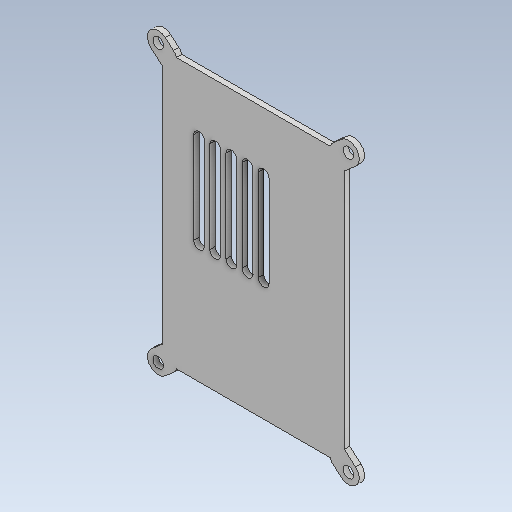
# Autodesk Inventor part: Case Cover Rev D
Saved by Autodesk Inventor 2021 (Build 250183000, 183)
## iProperties
Created: 2021-07-31
Part Number: Case Cover Rev D
Material: Generic
Document SubType Name: Modeling
Designer: cmzgt
Density: 1 g/cm^3
Appearance: Default
Author: cmzgt
Autodesk Inventor part; units mm, degrees
ref_plane "YZ Plane" through (0, 0, 0) normal (1, 0, 0) x (0, 1, 0)
ref_plane "XZ Plane" through (0, 0, 0) normal (0, 1, 0) x (-1, 0, 0)
ref_plane "XY Plane" through (0, 0, 0) normal (0, 0, 1) x (1, 0, 0)
sketch "Sketch1" plane through (0, 0, 0) normal (0, 0, 1) x (1, 0, 0)
  circle A0 centre (35.3094, -51.3621) radius 1.985 projected
  circle A1 centre (-35.3094, -51.3621) radius 1.985 projected
  circle A2 centre (-35.3094, 51.3621) radius 1.985 projected
  circle A3 centre (35.3094, 51.3621) radius 1.985 projected
  line L0 (28.5119, 50.05) -> (-28.5119, 50.05) projected
  arc A4 (-28.5119, 50.05) -> (-29.6663, 51.7567) centre (-32.2906, 48.7379) ccw projected
  line L1 (-32.6852, 54.381) -> (-29.6663, 51.7567) projected
  arc A5 (-32.6852, 54.381) -> (-37.9337, 48.3433) centre (-35.3094, 51.3621) ccw projected
  line L2 (-33.8, 44.7499) -> (-37.9337, 48.3433) projected
  line L3 (-33.8, 44.7499) -> (-33.8, -44.7499) projected
  line L4 (-37.9337, -48.3433) -> (-33.8, -44.7499) projected
  arc A6 (-37.9337, -48.3433) -> (-32.6852, -54.381) centre (-35.3094, -51.3621) ccw projected
  line L5 (-29.6663, -51.7567) -> (-32.6852, -54.381) projected
  arc A7 (-29.6663, -51.7567) -> (-28.5119, -50.05) centre (-32.2906, -48.7379) ccw projected
  line L6 (-28.5119, -50.05) -> (28.5119, -50.05) projected
  arc A8 (28.5119, -50.05) -> (29.6663, -51.7567) centre (32.2906, -48.7379) ccw projected
  line L7 (32.6852, -54.381) -> (29.6663, -51.7567) projected
  arc A9 (32.6852, -54.381) -> (37.9337, -48.3433) centre (35.3094, -51.3621) ccw projected
  line L8 (33.8, -44.7499) -> (37.9337, -48.3433) projected
  line L9 (33.8, -44.7499) -> (33.8, 44.7499) projected
  line L10 (37.9337, 48.3433) -> (33.8, 44.7499) projected
  arc A10 (37.9337, 48.3433) -> (32.6852, 54.381) centre (35.3094, 51.3621) ccw projected
  line L11 (29.6663, 51.7567) -> (32.6852, 54.381) projected
  arc A11 (29.6663, 51.7567) -> (28.5119, 50.05) centre (32.2906, 48.7379) ccw projected
  line L12 (-30.6, -44.85) -> (-30.6, 44.85) projected
  arc A12 (-28.6, 46.85) -> (-30.6, 44.85) centre (-28.6, 44.85) ccw projected
  line L13 (-28.6, 46.85) -> (28.6, 46.85) projected
  arc A13 (30.6, 44.85) -> (28.6, 46.85) centre (28.6, 44.85) ccw projected
  line L14 (30.6, 44.85) -> (30.6, -44.85) projected
  arc A14 (28.6, -46.85) -> (30.6, -44.85) centre (28.6, -44.85) ccw projected
  line L15 (28.6, -46.85) -> (-28.6, -46.85) projected
  arc A15 (-30.6, -44.85) -> (-28.6, -46.85) centre (-28.6, -44.85) ccw projected
  point P0 (0, 0)
extrude "Extrusion1" add sketch "Sketch1" along normal blind 2 contours A11 L11 A10 L10 L9 L8 A9 L7 A8 L6 A7 L5 A6 L4 L3 L2 A5 L1 A4 L0 | L12 A12 L13 A13 L14 A14 L15 A15
sketch "Sketch3" plane through (0, 0, 2) normal (0, 0, 1) x (1, 0, 0)
  line L0 (-5.7986, 18.4674) -> (8.3133, 18.4674) projected
  line L1 (8.3133, 18.4674) -> (8.3133, 4.4942) projected
  line L2 (8.3133, 4.4942) -> (-5.7986, 4.4942) projected
  line L3 (-5.7986, 4.4942) -> (-5.7986, 18.4674) projected
  line L4 (-8.1427, -5.5192) -> (-8.1427, 28.4808) construction
  line L5 (-6.1427, -5.5192) -> (-6.1427, 28.4808)
  line L6 (-10.1427, 28.4808) -> (-10.1427, -5.5192)
  arc A0 (-10.1427, -5.5192) -> (-6.1427, -5.5192) centre (-8.1427, -5.5192) ccw
  arc A1 (-6.1427, 28.4808) -> (-10.1427, 28.4808) centre (-8.1427, 28.4808) ccw
  arc A2 (-0.1427, 28.4808) -> (-4.1427, 28.4808) centre (-2.1427, 28.4808) ccw
  line L7 (-0.1427, -5.5192) -> (-0.1427, 28.4808)
  line L8 (-4.1427, 28.4808) -> (-4.1427, -5.5192)
  arc A3 (-4.1427, -5.5192) -> (-0.1427, -5.5192) centre (-2.1427, -5.5192) ccw
  line L9 (5.8573, -5.5192) -> (5.8573, 28.4808)
  arc A4 (5.8573, 28.4808) -> (1.8573, 28.4808) centre (3.8573, 28.4808) ccw
  line L10 (1.8573, 28.4808) -> (1.8573, -5.5192)
  arc A5 (1.8573, -5.5192) -> (5.8573, -5.5192) centre (3.8573, -5.5192) ccw
  line L11 (-16.1427, 28.4808) -> (-16.1427, -5.5192)
  arc A6 (-12.1427, 28.4808) -> (-16.1427, 28.4808) centre (-14.1427, 28.4808) ccw
  line L12 (-12.1427, -5.5192) -> (-12.1427, 28.4808)
  arc A7 (-16.1427, -5.5192) -> (-12.1427, -5.5192) centre (-14.1427, -5.5192) ccw
  line L13 (-22.1427, 28.4808) -> (-22.1427, -5.5192)
  arc A8 (-18.1427, 28.4808) -> (-22.1427, 28.4808) centre (-20.1427, 28.4808) ccw
  line L14 (-18.1427, -5.5192) -> (-18.1427, 28.4808)
  arc A9 (-22.1427, -5.5192) -> (-18.1427, -5.5192) centre (-20.1427, -5.5192) ccw
  point P0 (0, 0)
  point P1 (-8.1427, 11.4808)
  dimension "d8" = 17
  dimension "d9" = 4
  dimension "d12" = 6
  dimension "d19" = 6
  dimension "d26" = 6
  constraints: 24 end point, 20 point on circle, 10 centre point, 4 tangent, 3 horizontal, 1 midpoint, 1 parallel, 1 vertical, 40 other
  measures "d8" distance of point (-8.143, 11.481) L4.end
  measures "d9" diameter of A1
  measures "d12" distance of L4.end A2.centre
  measures "d19" distance of L7.start L9.start
  measures "d26" distance of L6.start L11.start
extrude "Extrusion3" cut sketch "Sketch3" against normal up to surface (2 mm away) contours L8 A2 L7 L0 | L0 L7 L2 L8 | L2 L7 A3 L8 | L10 A4 L9 L0 | L0 L9 L2 L10 | L2 L9 A5 L10 | A0 L6 A1 L5 | A6 L12 A7 L11 | A8 L14 A9 L13
body "Solid1"
